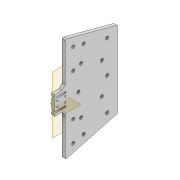
# Autodesk Inventor part: Foam_wing_mount_clamp_new
Saved by Autodesk Inventor 2022 (Build 260153000, 153)
## iProperties
Created: 2022-06-29
Part Number: Foam_wing_mount_clamp_new
Material: Generic
Document SubType Name: Modeling
Designer: dell
Density: 1 g/cm^3
Appearance: Default
Mass: 30.3471 g
Surface Area: 119.338 cm^2
Volume: 30.3471 cm^3
Author: dell
Autodesk Inventor part; units mm, degrees
ref_plane "YZ Plane" through (0, 0, 0) normal (1, 0, 0) x (0, 1, 0)
ref_plane "XZ Plane" through (0, 0, 0) normal (0, 1, 0) x (-1, 0, 0)
ref_plane "XY Plane" through (0, 0, 0) normal (0, 0, 1) x (1, 0, 0)
sketch "Sketch1" plane through (0, 0, 0) normal (0, 0, 1) x (1, 0, 0)
  line L0 (0, 0) -> (6, 0)
  line L1 (6, 0) -> (6, 100)
  line L2 (6, 100) -> (0, 100)
  line L3 (0, 100) -> (0, 0)
  dimension "d0" = 6
  dimension "d1" = 100
  constraints: 8 end point, 2 parallel, 1 horizontal, 1 perpendicular
  measures "d0" distance between parallel lines of L3 L1
  measures "d1" distance between parallel lines of L0 L2
extrude "Extrusion1" add sketch "Sketch1" along normal blind 5
sketch "Sketch3" plane through (0, 0, 5) normal (0, 0, 1) x (1, 0, 0)
  line L0 (6, 0) -> (6, 100) projected
  line L1 (6, 100) -> (0, 100) projected
  line L2 (0, 100) -> (0, 0) projected
  line L3 (0, 0) -> (6, 0) projected
  line L4 (0, 50) -> (6, 50) construction
  line L5 (6, 0) -> (6, 100) construction
  line L6 (0, 100) -> (0, 0) projected
  line L7 (0, 60) -> (6, 60)
  line L8 (6, 60) -> (6, 40)
  line L9 (6, 40) -> (0, 40)
  line L10 (0, 40) -> (0, 60)
  line L11 (0, 63.1) -> (6, 63.1)
  line L12 (6, 63.1) -> (6, 68.1)
  line L13 (6, 68.1) -> (0, 68.1)
  line L14 (0, 68.1) -> (0, 63.1)
  line L15 (0, 36.9) -> (6, 36.9)
  line L16 (6, 36.9) -> (6, 31.9)
  line L17 (6, 31.9) -> (0, 31.9)
  line L18 (0, 31.9) -> (0, 36.9)
  point P0 (0, 31.9)
  point P1 (6, 31.9)
  point P2 (6, 36.9)
  point P3 (0, 40)
  point P4 (6, 40)
  point P5 (6, 60)
  point P6 (6, 68.1)
  point P7 (0, 68.1)
  point P8 (6, 63.1)
  dimension "d6" = 50
  dimension "d7" = 100
  dimension "d8" = 10
  dimension "d9" = 10
  dimension "d10" = 5
  dimension "d11" = 3.1
  dimension "d12" = 3.1
  dimension "d13" = 5
  constraints: 26 end point, 6 parallel, 6 point on line, 4 perpendicular, 3 horizontal, 2 midpoint
  measures "d6" distance between parallel lines of L3 L4
  measures "d7" distance between parallel lines of L1 L3
  measures "d8" distance between parallel lines of L4 L9
  measures "d9" distance between parallel lines of L4 L7
  measures "d10" distance between parallel lines of L13 L11
  measures "d11" distance between parallel lines of L7 L11
  measures "d12" distance between parallel lines of L9 L15
  measures "d13" distance between parallel lines of L17 L15
extrude "Extrusion2" add sketch "Sketch3" along normal blind 20 contours L17 L2 L15 L0 | L9 L2 L7 L0 | L11 L2 L13 L0
ref_plane "Work Plane1" through (3, 0, 0) normal (1, 0, 0) x (0, 0, -1)
sketch "Sketch13" plane through (6, 0, 0) normal (1, 0, 0) x (0, 0, -1)
  circle A0 centre (-5, 55) radius 1.5
  circle A1 centre (-5, 45) radius 1.5
  circle A2 centre (-20, 55) radius 1.5
  circle A3 centre (-20, 45) radius 1.5
  line L0 (-5, 60) -> (-25, 60) projected
  line L1 (-5, 40) -> (-25, 40) projected
  line L2 (-25, 40) -> (-25, 60) projected
  line L3 (0, 0) -> (0, 100) projected
  dimension "d57" = 3
  dimension "d58" = 3
  dimension "d59" = 3
  dimension "d60" = 3
  dimension "d61" = 5
  dimension "d62" = 5
  dimension "d63" = 5
  dimension "d64" = 5
  dimension "d65" = 5
  dimension "d67" = 5
  dimension "d69" = 5
  dimension "d70" = 5
  constraints: 4 centre point
  measures "d57" diameter of A0
  measures "d58" diameter of A1
  measures "d59" diameter of A2
  measures "d60" diameter of A3
  measures "d61" distance from line of L0 A0.centre
  measures "d62" distance from line of L0 A2.centre
  measures "d63" distance from line of L1 A1.centre
  measures "d64" distance from line of L1 A3.centre
  measures "d65" distance from line of L2 A3.centre
  measures "d67" distance from line of A2.centre L2
  measures "d69" distance from line of L3 A1.centre
  measures "d70" distance from line of L3 A0.centre
extrude "Extrusion11" cut sketch "Sketch13" against normal blind 180
ref_plane "Work Plane3" through (0, 50, 5) normal (0, 1, 0) x (1, 0, 0)
thicken "Thicken1" operation add thickness 1 both sides no extend neighbours yes toward (0, 0, -1) faces at (2, 37.9333, 5)
thicken "Thicken2" operation add thickness 1 both sides no extend neighbours yes toward (0, 0, -1) faces at (2, 62.0667, 5)
sketch "Sketch14" plane through (6, 0, 0) normal (1, 0, 0) x (0, 0, -1)
  line L0 (-5, 68.1) -> (-5, 100) projected
  line L1 (-5, 100) -> (-5, 150)
  line L2 (0, 0) -> (-5, 0) projected
  line L3 (-5, 0) -> (-5, -50)
  line L4 (-5, -50) -> (295, 30)
  line L5 (295, 30) -> (295, 70)
  line L6 (295, 70) -> (-5, 150)
  circle A0 centre (-5, 45) radius 1.5 projected
  circle A1 centre (-5, 55) radius 1.5 projected
  circle A2 centre (-20, 45) radius 1.5 projected
  circle A3 centre (-20, 55) radius 1.5 projected
  line L7 (0, 0) -> (0, 100) projected
  line L8 (0, 100) -> (-5, 100) projected
  line L9 (-5, 68.1) -> (-5, 100) projected
  line L10 (-5, 68.1) -> (-25, 68.1) projected
  line L11 (-25, 63.1) -> (-25, 68.1) projected
  line L12 (-4, 63.1) -> (-25, 63.1) projected
  line L13 (-4, 60) -> (-4, 63.1) projected
  line L14 (-4, 60) -> (-25, 60) projected
  line L15 (-25, 40) -> (-25, 60) projected
  line L16 (-4, 40) -> (-25, 40) projected
  line L17 (-4, 36.9) -> (-4, 40) projected
  line L18 (-4, 36.9) -> (-25, 36.9) projected
  line L19 (-25, 31.9) -> (-25, 36.9) projected
  line L20 (-5, 31.9) -> (-25, 31.9) projected
  line L21 (-5, 0) -> (-5, 31.9) projected
  line L22 (0, 0) -> (-5, 0) projected
  dimension "d78" = 50
  dimension "d79" = 50
  dimension "d80" = 300
  dimension "d81" = 80
  dimension "d82" = 80
  constraints: 10 end point, 2 vertical, 1 parallel
  measures "d78" distance of L0.end L1.end
  measures "d79" distance of L3.end L2.end
  measures "d80" distance between parallel lines of L5 L3
  measures "d81" vertical distance of L1.end L5.end
  measures "d82" vertical distance of L3.end L4.end
extrude "Extrusion12" add sketch "Sketch14" against normal blind 6 contours L1 L6 L5 L4 L3 L2 L7 L8
sketch "Sketch15" plane through (6, 40, 25) normal (1, 0, 0) x (0, 0, -1)
  circle A0 centre (35, 90) radius 2.975
  line L0 (20, 28.1) -> (20, 110) projected
  circle A1 centre (170, 55) radius 2.975
  circle A2 centre (310, 20) radius 2.975
  circle A3 centre (100, 10) radius 2.975
  line L1 (-64.0657, 10) -> (384.394, 10) projected
  circle A4 centre (240, 10) radius 2.975
  circle A5 centre (100, 72) radius 2.975
  circle A6 centre (240, 37) radius 2.975
  circle A7 centre (35, 50) radius 2.975
  circle A8 centre (90, 40) radius 2.975
  circle A9 centre (55, 85) radius 2.975
  circle A10 centre (50, 55) radius 2.975
  circle A11 centre (45, 10) radius 2.975
  point P0 (25, -40)
  dimension "d85" = 5.95
  dimension "d86" = 15
  dimension "d87" = 20
  dimension "d88" = 5.95
  dimension "d89" = 150
  dimension "d90" = 55
  dimension "d91" = 5.95
  dimension "d92" = 290
  dimension "d93" = 90
  dimension "d96" = 5.95
  dimension "d97" = 80
  dimension "d98" = 5.95
  dimension "d99" = 220
  dimension "d104" = 5.95
  dimension "d105" = 80
  dimension "d106" = 38
  dimension "d107" = 5.95
  dimension "d108" = 220
  dimension "d109" = 73
  dimension "d110" = 5.95
  dimension "d111" = 15
  dimension "d112" = 40
  dimension "d115" = 5.95
  dimension "d116" = 30
  dimension "d117" = 70
  dimension "d118" = 5.95
  dimension "d119" = 35
  dimension "d120" = 75
  dimension "d121" = 5.95
  dimension "d122" = 30
  dimension "d123" = 45
  dimension "d124" = 5.95
  dimension "d125" = 25
  constraints: 12 centre point, 3 point on line
  measures "d85" diameter of A0
  measures "d86" distance from line of L0 A0.centre
  measures "d87" vertical distance of L0.end A0.centre
  measures "d88" diameter of A1
  measures "d89" distance from line of L0 A1.centre
  measures "d90" vertical distance of L0.end A1.centre
  measures "d91" diameter of A2
  measures "d92" distance from line of L0 A2.centre
  measures "d93" vertical distance of L0.end A2.centre
  measures "d96" diameter of A3
  measures "d97" distance from line of L0 A3.centre
  measures "d98" diameter of A4
  measures "d99" distance from line of L0 A4.centre
  measures "d104" diameter of A5
  measures "d105" distance from line of L0 A5.centre
  measures "d106" vertical distance of L0.end A5.centre
  measures "d107" diameter of A6
  measures "d108" distance from line of L0 A6.centre
  measures "d109" vertical distance of L0.end A6.centre
  measures "d110" diameter of A7
  measures "d111" distance from line of L0 A7.centre
  measures "d112" distance from line of L1 A7.centre
  measures "d115" diameter of A8
  measures "d116" distance from line of L1 A8.centre
  measures "d117" distance from line of L0 A8.centre
  measures "d118" diameter of A9
  measures "d119" distance from line of L0 A9.centre
  measures "d120" distance from line of L1 A9.centre
  measures "d121" diameter of A10
  measures "d122" distance from line of L0 A10.centre
  measures "d123" distance from line of L1 A10.centre
  measures "d124" diameter of A11
  measures "d125" distance from line of L0 A11.centre
extrude "Extrusion13" cut sketch "Sketch15" against normal blind 100
mirror "Mirror1" about plane through (0, 50, 5) normal (0, 1, 0) of "Extrusion13"
chamfer "Chamfer1" distance 6 angle 45 2 edges at (3, 68.1, 5) (3, 31.9, 5)
fillet "Fillet2" radius 2 4 edges at (3, 150, 5) (3, -50, 5) (3, 70, -295) (3, 30, -295)
fillet "Fillet3" radius 0.8 4 edges at (3, 63.1, 4) (3, 60, 4) (3, 36.9, 4) (3, 40, 4)
sketch "Sketch19" plane through (6, 40, 25) normal (1, 0, 0) x (0, 0, -1)
  circle A0 centre (50, -35) radius 2.975 projected
  circle A1 centre (240, -17) radius 2.975 projected
  circle A2 centre (170, -35) radius 2.975 projected
  circle A3 centre (35, -70) radius 2.975 projected
  circle A4 centre (100, -52) radius 2.975 projected
  circle A5 centre (55, -65) radius 2.975 projected
  circle A6 centre (90, -20) radius 2.975 projected
  circle A7 centre (310, 0) radius 2.975 projected
  circle A8 centre (35, -30) radius 2.975 projected
  circle A9 centre (50, 55) radius 2.975 projected
  circle A10 centre (240, 37) radius 2.975 projected
  circle A11 centre (170, 55) radius 2.975 projected
  circle A12 centre (35, 90) radius 2.975 projected
  circle A13 centre (100, 72) radius 2.975 projected
  circle A14 centre (55, 85) radius 2.975 projected
  circle A15 centre (90, 40) radius 2.975 projected
  circle A16 centre (240, 10) radius 2.975 projected
  circle A17 centre (310, 20) radius 2.975 projected
  circle A18 centre (100, 10) radius 2.975 projected
  circle A19 centre (35, 50) radius 2.975 projected
  circle A20 centre (45, 10) radius 2.975 projected
  circle A21 centre (20, 5) radius 1.5 projected
  circle A22 centre (20, 15) radius 1.5 projected
  circle A23 centre (5, 5) radius 1.5 projected
  circle A24 centre (5, 15) radius 1.5 projected
  arc A25 (318.5153, -10.3959) -> (320, -8.4634) centre (318, -8.4634) ccw projected
  line L0 (320, -8.4634) -> (320, 28.4634) projected
  arc A26 (320, 28.4634) -> (318.5153, 30.3959) centre (318, 28.4634) ccw projected
  line L1 (318.5153, 30.3959) -> (22.5153, 109.3292) projected
  arc A27 (22.5153, 109.3292) -> (20, 107.3968) centre (22, 107.3968) ccw projected
  line L2 (20, 34.1) -> (20, 107.3968) projected
  line L3 (14, 28.1) -> (20, 34.1) projected
  line L4 (14, 28.1) -> (0, 28.1) projected
  line L5 (0, 23.1) -> (0, 28.1) projected
  line L6 (20.2, 23.1) -> (0, 23.1) projected
  arc A28 (21, 22.3) -> (20.2, 23.1) centre (20.2, 22.3) ccw projected
  line L7 (21, 20.8) -> (21, 22.3) projected
  arc A29 (20.2, 20) -> (21, 20.8) centre (20.2, 20.8) ccw projected
  line L8 (20.2, 20) -> (0, 20) projected
  line L9 (0, 0) -> (0, 20) projected
  line L10 (20.2, 0) -> (0, 0) projected
  arc A30 (21, -0.8) -> (20.2, 0) centre (20.2, -0.8) ccw projected
  line L11 (21, -2.3) -> (21, -0.8) projected
  arc A31 (20.2, -3.1) -> (21, -2.3) centre (20.2, -2.3) ccw projected
  line L12 (20.2, -3.1) -> (0, -3.1) projected
  line L13 (0, -8.1) -> (0, -3.1) projected
  line L14 (14, -8.1) -> (0, -8.1) projected
  line L15 (20, -14.1) -> (14, -8.1) projected
  line L16 (20, -14.1) -> (20, -87.3968) projected
  arc A32 (20, -87.3968) -> (22.5153, -89.3292) centre (22, -87.3968) ccw projected
  line L17 (22.5153, -89.3292) -> (318.5153, -10.3959) projected
  line L18 (22.5153, 109.3292) -> (318.5153, 30.3959) projected
  line L19 (120, 83.3333) -> (120, -63.3333)
  line L20 (318.5153, -10.3959) -> (22.5153, -89.3292) projected
  point P0 (25, -40)
  dimension "d126" = 120
  constraints: 2 end point, 2 point on line, 1 vertical
  measures "d126" distance between parallel lines of L9 L19
extrude "Extrusion14" cut sketch "Sketch19" against normal blind 100 contours L17 L19 L1 A26 L0 A25
fillet "Fillet4" radius 2 2 edges at (3, -23.3333, -95) (3, 123.3333, -95)
equation "\"d6\" = 0.5 * d7"
equation "\"d62\" = d61"
equation "\"d63\" = d61"
equation "\"d64\" = d61"
equation "\"d67\" = d65"
equation "\"d69\" = d65"
equation "\"d70\" = d65"
body "Solid1"
